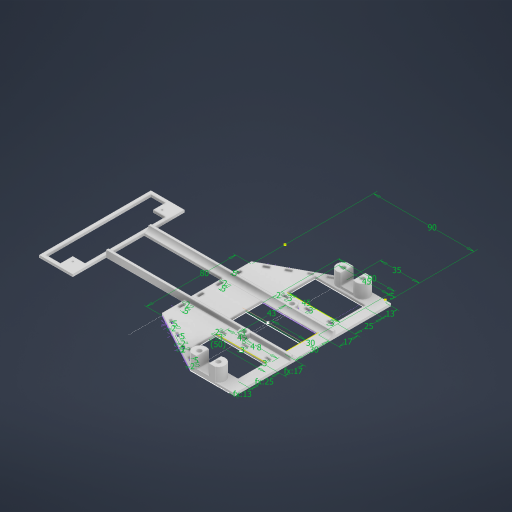
# Autodesk Inventor part: Part4
Saved by Autodesk Inventor 2023 (Build 270158000, 158)
## iProperties
Created: 2023-02-02
Part Number: Part4
Material: Generic
Document SubType Name: Modeling
Designer: aniela
Density: 1 g/cm^3
Appearance: Default
Author: aniela
Autodesk Inventor part; units mm, degrees
ref_plane "YZ Plane" through (0, 0, 0) normal (1, 0, 0) x (0, 1, 0)
ref_plane "XZ Plane" through (0, 0, 0) normal (0, 1, 0) x (-1, 0, 0)
ref_plane "XY Plane" through (0, 0, 0) normal (0, 0, 1) x (1, 0, 0)
sketch "Sketch1" plane through (0, 0, 0) normal (0, 1, 0) x (-1, 0, 0)
  line L0 (0, 0) -> (35, 0) construction
  line L1 (90, 30) -> (90, 110) construction
  line L2 (35, 140) -> (0, 140)
  line L3 (0, 140) -> (0, 0)
  line L4 (0, 0) -> (35, 0) construction
  line L5 (35, 0) -> (35, 140) construction
  line L6 (35, 140) -> (0, 140) construction
  line L7 (0, 140) -> (0, 0) construction
  line L8 (90, 110) -> (35, 140) construction
  line L9 (35, 0) -> (90, 30) construction
  line L10 (35, 140) -> (90, 110) construction
  line L11 (35, 0) -> (90, 30) construction
  line L12 (90, 110) -> (90, 30) construction
  line L13 (35, 0) -> (90, 30)
  line L14 (90, 30) -> (90, 110)
  line L15 (90, 110) -> (35, 140)
  line L16 (5, 127) -> (50, 127) construction
  line L17 (50, 127) -> (50, 102) construction
  line L18 (50, 102) -> (5, 102) construction
  line L19 (5, 102) -> (5, 127) construction
  line L20 (50, 127) -> (50, 102) construction
  line L21 (50, 102) -> (5, 102) construction
  line L22 (50, 127) -> (50, 102)
  line L23 (50, 127) -> (5, 127)
  line L24 (50, 102) -> (5, 102)
  line L25 (5, 102) -> (5, 127)
  line L26 (35, 0) -> (0, 0) construction
  line L27 (5, 13) -> (50, 13) construction
  line L28 (50, 13) -> (50, 38) construction
  line L29 (50, 38) -> (5, 38) construction
  line L30 (5, 38) -> (5, 13) construction
  line L31 (50, 38) -> (5, 38) construction
  line L32 (5, 38) -> (5, 13) construction
  line L33 (5, 13) -> (50, 13) construction
  line L34 (50, 13) -> (50, 38) construction
  line L35 (5, 13) -> (50, 13) construction
  line L36 (50, 13) -> (50, 38) construction
  line L37 (50, 38) -> (5, 38) construction
  line L38 (5, 38) -> (5, 13) construction
  line L39 (50, 38) -> (50, 13)
  line L40 (50, 13) -> (5, 13)
  line L41 (5, 13) -> (5, 38)
  line L42 (5, 38) -> (50, 38)
  line L43 (9.9818, 0) -> (0, 0) construction
  line L44 (0, 0) -> (0, 55) construction
  line L45 (0, 55) -> (9.9818, 55) construction
  line L46 (9.9818, 55) -> (9.9818, 0) construction
  line L47 (5, 55) -> (55, 55) construction
  line L48 (55, 55) -> (55, 92) construction
  line L49 (5, 92) -> (5, 55) construction
  line L50 (5, 92) -> (5, 55) construction
  line L51 (5, 55) -> (55, 55) construction
  line L52 (55, 55) -> (55, 92) construction
  line L53 (55, 92) -> (55, 55) construction
  line L54 (55, 55) -> (5, 55)
  line L55 (35, 0) -> (0, 0)
  line L56 (55, 55) -> (55, 85)
  line L57 (55, 85) -> (5, 85)
  line L58 (5, 55) -> (5, 85)
  line L59 (90, 30) -> (90, 0) construction
  line L60 (90, 110) -> (90, 140) construction
  line L61 (50, 97) -> (50, 99)
  line L62 (5, 99) -> (5, 97)
  line L63 (50, 41) -> (50, 43)
  line L64 (5, 43) -> (5, 41)
  line L65 (45, 97) -> (45, 99)
  line L66 (30, 99) -> (30, 97)
  line L67 (25, 97) -> (25, 99)
  line L68 (9.4183, 99) -> (9.4183, 97)
  line L69 (50, 97) -> (45, 97)
  line L70 (45, 99) -> (50, 99)
  line L71 (25, 97) -> (30, 97)
  line L72 (30, 99) -> (25, 99)
  line L73 (9.4183, 99) -> (5, 99)
  line L74 (5, 97) -> (9.4183, 97)
  line L75 (45, 43) -> (45, 41)
  line L76 (30, 43) -> (30, 41)
  line L77 (25, 41) -> (25, 43)
  line L78 (9.9818, 43) -> (9.9818, 41)
  line L79 (50, 43) -> (45, 43)
  line L80 (45, 41) -> (50, 41)
  line L81 (30, 41) -> (25, 41)
  line L82 (25, 43) -> (30, 43)
  line L83 (9.9818, 41) -> (5, 41)
  line L84 (5, 43) -> (9.9818, 43)
  line L85 (88, 98) -> (86, 98)
  line L86 (86, 98) -> (86, 93)
  line L87 (86, 93) -> (88, 93)
  line L88 (88, 93) -> (88, 98)
  line L89 (86, 81) -> (88, 81)
  line L90 (88, 81) -> (88, 76)
  line L91 (88, 76) -> (86, 76)
  line L92 (86, 76) -> (86, 81)
  line L93 (88, 64) -> (86, 64)
  line L94 (86, 64) -> (86, 59)
  line L95 (86, 59) -> (88, 59)
  line L96 (88, 59) -> (88, 64)
  line L97 (86, 47) -> (88, 47)
  line L98 (88, 47) -> (88, 42)
  line L99 (88, 42) -> (86, 42)
  line L100 (86, 42) -> (86, 47)
  line L101 (81.8068, 112.1072) -> (77.4173, 114.5014)
  line L102 (77.4173, 114.5014) -> (76.4596, 112.7456)
  line L103 (76.4596, 112.7456) -> (80.8491, 110.3514)
  line L104 (69.036, 119.3398) -> (68.0783, 117.584)
  line L105 (68.0783, 117.584) -> (63.6888, 119.9782)
  line L106 (63.6888, 119.9782) -> (64.6465, 121.734)
  line L107 (64.6465, 121.734) -> (69.036, 119.3398)
  line L108 (56.3597, 126.7853) -> (55.402, 125.0295)
  line L109 (55.402, 125.0295) -> (51.7103, 127.0432)
  line L110 (51.7103, 127.0432) -> (56.0998, 124.6489)
  line L111 (56.0998, 124.6489) -> (51.7103, 127.0432)
  line L112 (51.7103, 127.0432) -> (52.668, 128.799)
  line L113 (52.668, 128.799) -> (56.3597, 126.7853)
  line L114 (44.6114, 132.6044) -> (43.6537, 130.8486)
  line L115 (43.6537, 130.8486) -> (39.2642, 133.2429)
  line L116 (39.2642, 133.2429) -> (40.222, 134.9987)
  line L117 (40.222, 134.9987) -> (44.6114, 132.6044)
  line L118 (0, 70) -> (90, 70)
  line L119 (0, 140) -> (35, 140) construction
  line L120 (90, 110) -> (90, 30) construction
  line L121 (35, 0) -> (0, 0)
  line L122 (0, 0) -> (0, 140)
  line L123 (0, 140) -> (35, 140) construction
  line L124 (35, 0) -> (0, 0) construction
  line L125 (0, 0) -> (0, 140) construction
  line L126 (90, 30) -> (35, 0) construction
  line L127 (35, 0) -> (90, 30) construction
  line L128 (90, 30) -> (90, 110) construction
  line L129 (90, 110) -> (90, 30)
  line L130 (90, 30) -> (35, 0)
  line L131 (35, 140) -> (0, 140) construction
  line L132 (9.9818, 140) -> (0, 140) construction
  line L133 (0, 140) -> (0, 85) construction
  line L134 (0, 85) -> (9.9818, 85) construction
  line L135 (55, 85) -> (55, 48) construction
  line L136 (5, 48) -> (5, 85) construction
  line L137 (5, 48) -> (5, 85) construction
  line L138 (55, 85) -> (55, 48) construction
  line L139 (55, 48) -> (55, 85) construction
  line L140 (35, 140) -> (0, 140)
  line L141 (55, 85) -> (55, 55)
  line L142 (5, 85) -> (5, 55)
  line L143 (90, 30) -> (90, 0) construction
  line L144 (81.8068, 27.8928) -> (77.4173, 25.4986)
  line L145 (77.4173, 25.4986) -> (76.4596, 27.2544)
  line L146 (76.4596, 27.2544) -> (80.8491, 29.6486)
  line L147 (69.036, 20.6602) -> (68.0783, 22.416)
  line L148 (68.0783, 22.416) -> (63.6888, 20.0218)
  line L149 (63.6888, 20.0218) -> (64.6465, 18.266)
  line L150 (64.6465, 18.266) -> (69.036, 20.6602)
  line L151 (56.3597, 13.2147) -> (55.402, 14.9705)
  line L152 (55.402, 14.9705) -> (51.7103, 12.9568)
  line L153 (51.7103, 12.9568) -> (56.0998, 15.3511)
  line L154 (56.0998, 15.3511) -> (51.7103, 12.9568)
  line L155 (51.7103, 12.9568) -> (52.668, 11.201)
  line L156 (52.668, 11.201) -> (56.3597, 13.2147)
  line L157 (44.6114, 7.3956) -> (43.6537, 9.1514)
  line L158 (43.6537, 9.1514) -> (39.2642, 6.7571)
  line L159 (39.2642, 6.7571) -> (40.222, 5.0013)
  line L160 (40.222, 5.0013) -> (44.6114, 7.3956)
  line L161 (81.8068, 27.8928) -> (80.8491, 29.6486)
  line L162 (80.8491, 110.3514) -> (81.8068, 112.1072)
  point P0 (27.5, 102)
  point P1 (27.5, 99)
  point P2 (7.2091, 99)
  point P3 (47.5, 99)
  point P4 (27.5, 38)
  point P5 (27.5, 41)
  point P6 (7.4909, 41)
  point P7 (90, 98)
  point P8 (81.75, 114.5)
  point P9 (82.8477, 113.9013)
  point P10 (78.5969, 116.2199)
  point P11 (70.3953, 120.6935)
  point P12 (57.0441, 127.9759)
  point P13 (57.0441, 127.9759)
  point P14 (82.8477, 26.0987)
  point P15 (78.5969, 23.7801)
  point P16 (70.3953, 19.3065)
  dimension "d144" = 13
  dimension "d145" = 25
  dimension "d146" = 17
  dimension "d147" = 30
  dimension "d148" = 17
  dimension "d149" = 25
  dimension "d150" = 13
  dimension "d151" = 5
  dimension "d152" = 45
  dimension "d153" = 50
  dimension "d157" = 80
  dimension "d158" = 35
  dimension "d159" = 90
  dimension "d213" = 50
  dimension "d214" = 2
  dimension "d215" = 45
  dimension "d216" = 2
  dimension "d217" = 45
  dimension "d218" = 3
  dimension "d219" = 3
  dimension "d220" = 3
  dimension "d221" = 3
  dimension "d222" = 3
  dimension "d223" = 3
  dimension "d224" = 2
  dimension "d225" = 5
  dimension "d227" = 2
  dimension "d228" = 5
  dimension "d229" = 5
  dimension "d230" = 5
  dimension "d231" = 2
  dimension "d232" = 2
  dimension "d233" = 5
  dimension "d234" = 2
  dimension "d235" = 5
  dimension "d236" = 5
  dimension "d237" = 2
  constraints: 326 end point, 41 symmetric about line, 38 parallel, 36 point on line, 26 collinear, 26 perpendicular, 14 horizontal, 9 midpoint, 8 equal length, 1 coincident, 1 vertical
  measures "d144" distance between parallel lines of L0 L27
  measures "d145" distance between parallel lines of L27 L29
  measures "d146" distance between parallel lines of L29 L47
  measures "d147" distance of L47.start L57.end
  measures "d148" distance between parallel lines of L57 L18
  measures "d149" distance between parallel lines of L18 L16
  measures "d150" distance between parallel lines of L16 L2
  measures "d151" distance between parallel lines of L32 L3
  measures "d152" distance between parallel lines of L30 L28
  measures "d153" distance between parallel lines of L58 L52
  measures "d157" distance of L1.start L1.end
  measures "d158" distance of L0.start L4.end
  measures "d159" distance between parallel lines of L3 L12
  measures "d213" distance from line of L17.end L3
  measures "d214" distance of L61.end L61.start
  measures "d215" distance of L62.end L61.start
  measures "d216" distance of L63.end L63.start
  measures "d217" distance of L64.end L63.start
  measures "d218" distance of point (27.5, 102) point (27.5, 99)
  measures "d219" distance from line of L18 point (7.209, 99)
  measures "d220" distance from line of L18 point (47.5, 99)
  measures "d221" distance of point (27.5, 38) point (27.5, 41)
  measures "d222" distance between parallel lines of L31 L80
  measures "d223" distance from line of L29 point (7.491, 41)
  measures "d224" distance of L87.end L86.end
  measures "d225" distance of L86.end L85.end
  measures "d227" distance of L95.end L94.end
  measures "d228" distance of L94.end L93.end
  measures "d229" distance of L97.end L98.end
  measures "d230" distance of L101.start L101.end
  measures "d231" distance of L101.end L102.end
  measures "d232" distance of L104.start L104.end
  measures "d233" distance of L104.end L105.end
  measures "d234" distance of L108.start L108.end
  measures "d235" distance of L109.end L110.end
  measures "d236" distance of L114.end L115.end
  measures "d237" distance of L115.end L116.end
sketch "Sketch2" plane through (0, 0, 0) normal (0, 1, 0) x (-1, 0, 0)
  point P0 (0, 0)
sketch "Sketch3" plane through (0, 0, 0) normal (0, 1, 0) x (-1, 0, 0)
  point P0 (0, 0)
sketch "Sketch4" plane through (0, 0, 0) normal (0, 1, 0) x (-1, 0, 0)
  line L0 (0, 0) -> (35.5492, 0)
  line L1 (0, 0) -> (35, 0) construction
  line L2 (35, 0) -> (90, 30) construction
  line L3 (35, 0) -> (0, 0)
  constraints: 4 end point, 2 horizontal
extrude "Extrusion1" add sketch "Sketch1" along normal blind 2 contours L15 L14 L118 L56 L57 L58 L3 L2 | L118 L58 L54 L56 L14 L13 L55 L3
sketch "Sketch5" plane through (0, 2, 0) normal (0, 1, 0) x (1, 0, 0)
  line L0 (0, 0) -> (-35, 0) projected
  line L1 (-15, 0) -> (-32, 0)
  line L2 (-32, 0) -> (-32, -11)
  line L3 (-32, -11) -> (-15, -11)
  line L4 (-15, -11) -> (-15, 0)
  line L5 (-32, 0) -> (-15, 0)
  line L6 (-15, 0) -> (-15, -11)
  line L7 (-15, -11) -> (-32, -11)
  line L8 (-32, -11) -> (-32, 0)
  line L9 (-35, -140) -> (0, -140) projected
  line L10 (-15, -140) -> (-32, -140)
  line L11 (-32, -140) -> (-32, -129)
  line L12 (-32, -129) -> (-15, -129)
  line L13 (-15, -129) -> (-15, -140)
  line L14 (-32, -129) -> (-15, -129)
  line L15 (-15, -129) -> (-15, -140)
  line L16 (-15, -140) -> (-32, -140)
  line L17 (-32, -140) -> (-32, -129)
  dimension "d22" = 17
  dimension "d23" = 11
  dimension "d24" = 11
  constraints: 32 end point, 8 parallel, 4 horizontal, 4 perpendicular, 4 point on line
  measures "d22" distance of L3.end L2.end
  measures "d23" distance of L2.end L1.end
  measures "d24" distance of L10.end L11.end
extrude "Extrusion2" add sketch "Sketch5" along normal blind 2
sketch "Sketch6" plane through (0, 4, 0) normal (0, 1, 0) x (1, 0, 0)
  line L0 (-32, 0) -> (-32, -11) projected
  line L1 (-32, 0) -> (-29, 0)
  line L2 (-29, 0) -> (-29, -11)
  line L3 (-29, -11) -> (-32, -11)
  line L4 (-32, -11) -> (-32, 0)
  line L5 (-15, -11) -> (-15, 0) projected
  line L6 (-32, -11) -> (-15, -11) projected
  line L7 (-15, 0) -> (-18, 0)
  line L8 (-18, 0) -> (-18, -11)
  line L9 (-18, -11) -> (-15, -11)
  line L10 (-15, -11) -> (-15, 0)
  line L11 (-32, -11) -> (-32, 0)
  line L12 (0, 0) -> (-35, 0) projected
  line L13 (-32, -11) -> (-15, -11)
  line L14 (-32, 0) -> (-15, 0)
  line L15 (-15, -129) -> (-15, -140) projected
  line L16 (-32, -129) -> (-15, -129) projected
  line L17 (-15, -140) -> (-18, -140)
  line L18 (-18, -140) -> (-18, -129)
  line L19 (-18, -129) -> (-15, -129)
  line L20 (-15, -129) -> (-15, -140)
  line L21 (-32, -129) -> (-29, -129)
  line L22 (-29, -129) -> (-29, -140)
  line L23 (-29, -140) -> (-32, -140)
  line L24 (-32, -140) -> (-32, -129)
  line L25 (-35, -140) -> (-32, -140) projected
  line L26 (-32, -140) -> (-32, -129)
  line L27 (-32, -129) -> (-15, -129)
  line L28 (-18, -129) -> (-18, -140)
  line L29 (-35, -140) -> (0, -140) projected
  line L30 (-29, -129) -> (-29, -140)
  dimension "d27" = 3
  dimension "d28" = 3
  constraints: 46 end point, 11 equal length, 8 perpendicular, 4 horizontal, 4 point on line
  measures "d27" distance of L2.end L3.end
  measures "d28" distance of L9.end L8.end
extrude "Extrusion3" add sketch "Sketch6" along normal blind 10 contours L15 L17 L18 L16 | L22 L23 L24 L16
sketch "Sketch7" plane through (0, 4, 0) normal (0, 1, 0) x (1, 0, 0)
  line L0 (-15, -11) -> (-15, 0) projected
  line L1 (-32, -11) -> (-15, -11) projected
  line L2 (-15, 0) -> (-18, 0)
  line L3 (-18, 0) -> (-18, -11)
  line L4 (-18, -11) -> (-15, -11)
  line L5 (-15, -11) -> (-15, 0)
  line L6 (-18, -11) -> (-15, -11)
  line L7 (-15, -11) -> (-15, 0)
  line L8 (-15, 0) -> (-18, 0)
  line L9 (-18, 0) -> (-18, -11)
  line L10 (-32, 0) -> (-32, -11) projected
  line L11 (-32, 0) -> (-29, 0)
  line L12 (-29, 0) -> (-29, -11)
  line L13 (-29, -11) -> (-32, -11)
  line L14 (-32, -11) -> (-32, 0)
  line L15 (-18, -11) -> (-29, -11)
  point P0 (0, 0)
  dimension "d31" = 3
  dimension "d32" = 3
  constraints: 26 end point, 6 parallel, 4 perpendicular, 3 horizontal, 2 point on line
  measures "d31" distance of L4.end L3.end
  measures "d32" distance of L12.end L13.end
extrude "Extrusion4" add sketch "Sketch7" along normal blind 10
sketch "Sketch8" plane through (0, 2, 0) normal (0, 1, 0) x (1, 0, 0)
  line L0 (-80, -55) -> (-70, -55)
  line L1 (-70, -55) -> (-70, -85)
  line L2 (-70, -85) -> (-80, -85)
  line L3 (-80, -85) -> (-80, -55)
  circle A0 centre (-75, -60) radius 1.5
  circle A1 centre (-75, -80) radius 1.5
  point P0 (0, 0)
  dimension "d35" = 10
  dimension "d36" = 30
  dimension "d37" = 3
  dimension "d38" = 3
  constraints: 8 end point, 2 centre point, 2 parallel, 1 horizontal, 1 perpendicular
  measures "d35" distance of L1.end L2.end
  measures "d36" distance of L0.end L1.end
  measures "d37" diameter of A0
  measures "d38" diameter of A1
extrude "Extrusion5" cut sketch "Sketch8" along normal blind 2
sketch "Sketch11" plane through (0, 14, 0) normal (0, 1, 0) x (1, 0, 0)
  line L0 (-15, 0) -> (-15, -11) projected
  circle A0 centre (-15, -5.5) radius 3
  line L1 (-32, -11) -> (-32, 0) projected
  circle A1 centre (-32, -5.5) radius 3
  point P0 (0, 0)
  point P1 (-15, -2.5)
  point P2 (-15, -8.5)
  point P3 (-32, -2.5)
  point P4 (-32, -8.5)
  dimension "d55" = 6
  dimension "d56" = 6
  constraints: 2 centre point, 2 midpoint
  measures "d55" diameter of A0
  measures "d56" diameter of A1
extrude "Extrusion6" add sketch "Sketch11" against normal blind 12 contours A0 L0 | A1 L1 picked at (-13.8765, -5.0912) picked at (-33.7524, -6.0681)
sketch "Sketch12" plane through (0, 14, 0) normal (0, 1, 0) x (1, 0, 0)
  arc A0 (-15, -8.5) -> (-15, -2.5) centre (-15, -5.5) ccw projected
  circle A1 centre (-15, -5.5) radius 2
  point P0 (0, 0)
  dimension "d59" = 4
  constraints: 1 centre point, 1 coincident
  measures "d59" diameter of A1
sketch "Sketch13" plane through (0, 14, 0) normal (0, 1, 0) x (1, 0, 0)
  arc A0 (-32, -2.5) -> (-32, -8.5) centre (-32, -5.5) ccw projected
  circle A1 centre (-32, -5.5) radius 2
  point P0 (0, 0)
  dimension "d60" = 4
  constraints: 1 centre point, 1 coincident
  measures "d60" diameter of A1
hole "Hole3" at (-32, 14, 5.5) direction (0, -1, 0) diameter 3 end through all
hole "Hole4" at (-15, 14, 5.5) direction (0, -1, 0) diameter 3 end through all
sketch "Sketch14" plane through (0, 0, 0) normal (0, -1, 0) x (1, 0, 0)
  circle A0 centre (-15, 5.5) radius 1.5 projected
  circle A1 centre (-15, 5.5) radius 2
  circle A2 centre (-32, 5.5) radius 1.5 projected
  circle A3 centre (-32, 5.5) radius 2
  circle A4 centre (-15, 5.5) radius 2
  point P0 (0, 0)
  constraints: 3 centre point, 3 coincident, 1 concentric
extrude "Extrusion7" add sketch "Sketch14" against normal blind 3 contours A0 | A2
sketch "Sketch15" plane through (0, 14, 0) normal (0, 1, 0) x (1, 0, 0)
  line L0 (-15, -140) -> (-15, -129) projected
  arc A0 (-12.6021, -140) -> (-17.3979, -140) centre (-15, -134.5) ccw
  line L1 (-18, -129) -> (-18, -140) projected
  line L2 (-15, -140) -> (0, -140) projected
  line L3 (-18, -140) -> (-15, -140) projected
  arc A1 (-29, -129.3038) -> (-34.3979, -140) centre (-32, -134.5) ccw
  line L4 (-32, -129) -> (-32, -140) projected
  line L5 (-29, -140) -> (-18, -140) projected
  line L6 (-32, -140) -> (-29, -140) projected
  line L7 (-35, -140) -> (-32, -140) projected
  line L8 (-90, -110) -> (-35, -140) projected
  line L9 (-29, -140) -> (-29, -129) projected
  point P0 (0, 0)
  point P1 (-29.6021, -140)
  point P2 (-18, -129.3038)
  point P3 (-18, -139.6962)
  dimension "d138" = 12
  dimension "d139" = 12
  constraints: 5 point on line, 4 point on circle, 3 midpoint, 2 centre point, 1 horizontal alignment
  measures "d138" diameter of A0
  measures "d139" diameter of A1
extrude "Extrusion8" add sketch "Sketch15" against normal blind 12 contours L2 L3 A0 L1 | L9 L6 L7 A1
sketch "Sketch19" plane through (0, 0, 0) normal (0, -1, 0) x (1, 0, 0)
  point P0 (0, 0)
sketch "Sketch20" plane through (0, 14, 0) normal (0, 1, 0) x (1, 0, 0)
  circle A0 centre (-32, -134.5) radius 2 projected
  circle A1 centre (-32, -134.5) radius 2
  circle A2 centre (-15, -134.5) radius 2 projected
  circle A3 centre (-15, -134.5) radius 2
  point P0 (0, 0)
  constraints: 2 centre point, 2 coincident
extrude "Extrusion10" add sketch "Sketch20" against normal up to surface (14 mm away)
sketch "Sketch21" plane through (0, 0, 0) normal (0, -1, 0) x (1, 0, 0)
  point P0 (0, 0)
sketch "Sketch22" plane through (0, 14, 0) normal (0, 1, 0) x (1, 0, 0)
  arc A0 (-12.6021, -140) -> (-17.3979, -129) centre (-15, -134.5) ccw projected
  circle A1 centre (-15, -134.5) radius 1.5
  arc A2 (-32, -131.4998) -> (-32, -137.5002) centre (-32, -134.5) ccw projected
  circle A3 centre (-32, -134.5) radius 1.5
  point P0 (0, 0)
  point P1 (-15, -137.5)
  point P2 (-15, -131.5)
  dimension "d100" = 3
  dimension "d101" = 3
  constraints: 2 centre point, 2 coincident
  measures "d100" diameter of A1
  measures "d101" diameter of A3
extrude "Extrusion11" cut sketch "Sketch22" against normal blind 12
sketch "Sketch23" plane through (0, 14, 0) normal (0, 1, 0) x (1, 0, 0)
  arc A0 (-32, -131.4998) -> (-32, -137.5002) centre (-32, -134.5) ccw projected
  circle A1 centre (-32, -134.5) radius 1.5
  point P0 (0, 0)
  dimension "d104" = 3
  constraints: 1 centre point, 1 coincident
  measures "d104" diameter of A1
extrude "Extrusion12" cut sketch "Sketch23" against normal blind 12
sketch "Sketch24" plane through (0, 2, 0) normal (0, 1, 0) x (1, 0, 0)
  point P0 (0, 0)
sketch "Sketch25" plane through (0, 2, 0) normal (0, 1, 0) x (1, 0, 0)
  line L0 (-90, -110) -> (-35, -140) projected
  line L1 (-90, -30) -> (-90, -110) projected
  line L2 (-90, -90) -> (-90, -50)
  line L3 (-90, -50) -> (-160, -50)
  line L4 (-160, -50) -> (-160, -90)
  line L5 (-160, -90) -> (-91.3182, -90)
  line L6 (-91.3182, -90) -> (-90, -90)
  line L7 (-90, -84) -> (-160, -84)
  line L8 (-90, -56) -> (-160, -56)
  point P0 (0, 0)
  dimension "d117" = 40
  dimension "d118" = 70
  constraints: 14 end point, 6 perpendicular, 6 point on line
  measures "d117" distance of L2.start L2.end
  measures "d118" distance of L2.end L3.end
extrude "Extrusion13" add sketch "Sketch25" against normal blind 2 contours L1 L8 L4 L3 | L1 L6 L5 L4 L7
sketch "Sketch26" plane through (0, 2, 0) normal (0, 1, 0) x (1, 0, 0)
  line L0 (-160, -90) -> (-160, -84) projected
  line L1 (-160, -90) -> (-90, -90)
  line L2 (-90, -90) -> (-90, -88)
  line L3 (-90, -88) -> (-160, -88)
  line L4 (-160, -88) -> (-160, -90)
  line L5 (-90, -30) -> (-90, -50) projected
  line L6 (-160, -56) -> (-160, -50) projected
  line L7 (-90, -50) -> (-160, -50)
  line L8 (-160, -50) -> (-160, -52)
  line L9 (-160, -52) -> (-90, -52)
  line L10 (-90, -52) -> (-90, -50)
  point P0 (0, 0)
  dimension "d121" = 2
  dimension "d122" = 2
  constraints: 16 end point, 4 parallel, 2 horizontal, 2 perpendicular, 1 collinear, 1 point on line
  measures "d121" distance of L2.end L1.end
  measures "d122" distance of L8.end L7.end
extrude "Extrusion14" add sketch "Sketch26" along normal blind 4
fillet "Fillet5" radius 4 1 edges at (-125, 2, 52)
fillet "Fillet6" radius 4 1 edges at (-125, 2, 88)
sketch "Sketch27" plane through (0, 2, 0) normal (0, 1, 0) x (1, 0, 0)
  line L0 (-160, -50) -> (-90, -50) projected
  line L1 (-90, -90) -> (-160, -90) projected
  line L2 (-190, -120) -> (-160, -120)
  line L3 (-160, -120) -> (-160, -20)
  line L4 (-160, -20) -> (-190, -20)
  line L5 (-190, -20) -> (-190, -120)
  line L6 (-160, -117) -> (-190, -117)
  line L7 (-190, -117) -> (-190, -120)
  line L8 (-190, -120) -> (-160, -120)
  line L9 (-160, -120) -> (-160, -117)
  line L10 (-190, -117) -> (-187, -117)
  line L11 (-187, -117) -> (-187, -20)
  line L12 (-187, -20) -> (-190, -20)
  line L13 (-190, -20) -> (-190, -117)
  line L14 (-160, -20) -> (-190, -20)
  line L15 (-190, -20) -> (-190, -23)
  line L16 (-190, -23) -> (-160, -23)
  line L17 (-160, -23) -> (-160, -20)
  line L18 (-160, -20) -> (-163, -20)
  line L19 (-163, -20) -> (-163, -120)
  line L20 (-163, -120) -> (-160, -120)
  line L21 (-160, -120) -> (-160, -20)
  line L22 (-160, -106) -> (-174, -106)
  line L23 (-174, -106) -> (-174, -120)
  line L24 (-174, -120) -> (-160, -120)
  line L25 (-160, -120) -> (-160, -106)
  line L26 (-160, -20) -> (-174, -20)
  line L27 (-174, -20) -> (-174, -34)
  line L28 (-174, -34) -> (-160, -34)
  line L29 (-160, -34) -> (-160, -20)
  line L30 (-160, -56) -> (-160, -50) projected
  point P0 (0, 0)
  point P1 (-190, -120)
  point P2 (-187, -23)
  point P3 (-174, -23)
  point P4 (-163, -34)
  point P5 (-163, -106)
  point P6 (-174, -117)
  dimension "d127" = 3
  dimension "d128" = 3
  dimension "d129" = 3
  dimension "d130" = 14
  dimension "d131" = 14
  dimension "d209" = 30
  constraints: 56 end point, 14 parallel, 7 horizontal, 7 perpendicular, 7 point on line, 1 coincident, 1 collinear
  measures "d127" distance of L12.end L11.end
  measures "d128" distance of L15.end L14.end
  measures "d129" distance of L20.end L19.end
  measures "d130" distance of L24.end L23.end
  measures "d131" distance of L27.end L26.end
  measures "d209" distance of L3.end L4.end
extrude "Extrusion15" add sketch "Sketch27" against normal blind 2 contours L5 L6 L23 L2 | L23 L6 L19 L2 | L5 L16 L11 L6 | L19 L6 L3 L2 | L23 L22 L19 L6 | L5 L4 L11 L16 | L19 L22 L3 L6 | L11 L4 L27 L16 | L19 L28 L3 L22 | L27 L4 L19 L16 | L16 L19 L28 L27 | L19 L16 L3 L28 | L19 L4 L3 L16
sketch "Sketch28" plane through (0, 2, 0) normal (0, 1, 0) x (1, 0, 0)
  line L0 (-160, -20) -> (-160, -120) projected
  circle A0 centre (-170, -30) radius 0.75
  line L1 (-160, -20) -> (-160, -120) projected
  circle A1 centre (-170, -110) radius 0.75
  point P0 (0, 0)
  point P1 (-160, -38.6603)
  point P2 (-160, -50)
  point P3 (-160, -180)
  point P4 (-160, -90)
  dimension "d134" = 1.5
  dimension "d135" = 1.5
  dimension "d211" = 10
  dimension "d212" = 10
  constraints: 3 coincident, 2 centre point, 2 point on line
  measures "d134" diameter of A0
  measures "d135" diameter of A1
  measures "d211" distance from line of L0 A0.centre
  measures "d212" distance from line of L0 A1.centre
extrude "Extrusion16" cut sketch "Sketch28" against normal blind 2
ref_plane "Work Plane1" through (-55, 2, 70) normal (0, 0, -1) x (1, 0, 0)
mirror "Mirror1" about plane through (-55, 2, 70) normal (0, 0, -1) of "Extrusion8", "Extrusion11"
sketch "Sketch29" plane through (0, 2, 0) normal (0, 1, 0) x (1, 0, 0)
  circle A0 centre (-170, -30) radius 0.75 projected
  circle A1 centre (-170, -30) radius 0.5
  circle A2 centre (-200, -109.9594) radius 1.5
  point P0 (0, 0)
  dimension "d140" = 1
  dimension "d141" = 3
  constraints: 2 centre point, 1 coincident
  measures "d140" diameter of A1
  measures "d141" diameter of A2
extrude "Extrusion17" cut sketch "Sketch29" against normal blind 1 contours A1 | A2
sketch "Sketch30" plane through (0, 2, 0) normal (0, 1, 0) x (1, 0, 0)
  point P0 (0, 0)
sketch "Sketch31" plane through (0, 2, 0) normal (0, 1, 0) x (1, 0, 0)
  line L0 (-35, -91.5) -> (-35, -48.5) construction
  line L1 (-5, -55) -> (-5, -85) projected
  line L2 (-35, -91.5) -> (-35, -102) construction
  line L3 (-50, -102) -> (-5, -102) projected
  line L4 (-35, -48.5) -> (-35, -38) construction
  line L5 (-5, -38) -> (-50, -38) projected
  circle A0 centre (-35, -91.5) radius 2
  circle A1 centre (-35, -48.5) radius 2
  circle A2 centre (-35, -91.5) radius 4
  circle A3 centre (-35, -48.5) radius 4
  point P0 (0, 0)
  point P1 (-35, -70)
  dimension "d160" = 43
  dimension "d161" = 30
  dimension "d162" = 4
  dimension "d163" = 8
  constraints: 6 coincident, 6 end point, 4 centre point, 3 point on line, 2 vertical, 1 collinear, 1 midpoint
  measures "d160" distance of L0.start L0.end
  measures "d161" distance from line of L1 point (-35, -70)
  measures "d162" diameter of A0
  measures "d163" diameter of A2
extrude "Extrusion18" add sketch "Sketch31" along normal blind 4 contours A0 | A1 | A2 | A3
hole "Hole7" at (-35, 2, 91.5) at (-35, 2, 48.5) direction (0, 1, 0) diameter 4 depth 19.05 tip angle 118
hole "Hole8" at (-35, 2, 91.5) at (-35, 2, 48.5) direction (0, -1, 0) diameter 4 depth 19.05 tip angle 118
sketch "Sketch32" plane through (-90, 2, 90) normal (1, 0, 0) x (0, 0, -1)
  line L0 (0, 4) -> (0, 0)
  line L1 (-50, 0) -> (90, 0) projected
  line L2 (0, 4) -> (2, 4) projected
  line L3 (0, 4) -> (2, 4)
  arc A0 (2, 4) -> (5.993, 0) centre (5.993, 3.993) ccw
  line L4 (0, 0) -> (0, 4) projected
  line L5 (0, 0) -> (5.993, 0)
  point P0 (90, -2)
  constraints: 6 end point, 2 collinear, 2 point on circle, 2 point on line, 2 tangent, 1 centre point, 1 vertical
extrude "Extrusion19" add sketch "Sketch32" along normal blind 95
sketch "Sketch33" plane through (-90, 2, 50) normal (1, 0, 0) x (0, 0, -1)
  point P0 (50, -2)
sketch "Sketch34" plane through (-90, 2, 50) normal (1, 0, 0) x (0, 0, -1)
  point P0 (50, -2)
sketch "Sketch35" plane through (-90, 2, 50) normal (1, 0, 0) x (0, 0, -1)
  point P0 (50, -2)
sketch "Sketch36" plane through (-90, 2, 50) normal (1, 0, 0) x (0, 0, -1)
  line L0 (-2, 4) -> (0, 4) projected
  line L1 (-2, 4) -> (0, 4)
  line L2 (0, 0) -> (0, 4) projected
  line L3 (0, 4) -> (0, 0)
  arc A0 (-6, 0) -> (-2, 4) centre (-6, 4) ccw projected
  arc A1 (-6, 0) -> (-2, 4) centre (-6, 4) ccw
  line L4 (0, 0) -> (-6, 0)
  line L5 (-2.5, 0) -> (5.5, 0) projected
  line L6 (0, 0) -> (-6, 0) projected
  line L7 (-6, 0) -> (0, 0)
  point P0 (50, -2)
  constraints: 8 end point, 3 point on circle, 2 perpendicular, 2 tangent, 1 centre point, 1 collinear, 1 horizontal
extrude "Extrusion20" add sketch "Sketch36" along normal blind 95
hole "Hole9" at (-35, 2, 91.5) direction (0, 1, 0) diameter 4 depth 19.05 tip angle 118
hole "Hole10" at (-35, 2, 48.5) direction (0, 1, 0) diameter 4 depth 19.05 tip angle 118
sketch "Szkic37" plane through (0, 14, 0) normal (0, 1, 0) x (1, 0, 0)
  circle A0 centre (-32, -5.5) radius 1.5 projected
  circle A1 centre (-32, -5.5) radius 2
  circle A2 centre (-15, -5.5) radius 1.5 projected
  circle A3 centre (-15, -5.5) radius 2
  circle A4 centre (-32, -134.5) radius 1.5 projected
  circle A5 centre (-32, -134.5) radius 2
  circle A6 centre (-15, -134.5) radius 2
  point P0 (0, 0)
  dimension "d198" = 4
  dimension "d199" = 4
  dimension "d200" = 4
  dimension "d201" = 4
  constraints: 4 centre point, 3 coincident
  measures "d198" diameter of A1
  measures "d199" diameter of A3
  measures "d200" diameter of A5
  measures "d201" diameter of A6
hole "Otwór11" at (-32, 14, 5.5) at (-15, 14, 5.5) at (-15, 14, 134.5) at (-32, 14, 134.5) direction (0, -1, 0) diameter 4 depth 12 tip angle 118
sketch "Szkic38" plane through (0, 0, 140) normal (1, 0, 0) x (0, 0, -1)
  line L0 (0, 0) -> (0, 2) projected
  line L1 (0, 0) -> (140, 0) projected
  line L2 (0, 2) -> (140, 2)
  line L3 (140, 2) -> (140, 0)
  line L4 (140, 0) -> (0, 0)
  line L5 (0, 0) -> (0, 2)
  constraints: 8 end point, 2 parallel, 1 horizontal, 1 perpendicular
extrude "Wyciągnięcie proste21" add sketch "Szkic38" along normal blind 5
body "Solid1"
